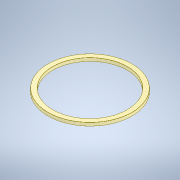
# Autodesk Inventor part: 201555-1-1-test
Saved by Autodesk Inventor 2021 (Build 250183000, 183)
## iProperties
Created: 2020-06-29
Part Number: 201555-1-1-test
Material: Nylon 6/6
Document SubType Name: Modeling
Density: 1.13 g/cm^3
Appearance: Nylon 6
Mass: 19.7025 g
Surface Area: 104.615 cm^2
Volume: 17.4358 cm^3
Author: MK
Subject: 100/120*5
Autodesk Inventor part; units mm, degrees
ref_plane "YZ Plane" through (0, 0, 0) normal (1, 0, 0) x (0, 1, 0)
ref_plane "XZ Plane" through (0, 0, 0) normal (0, 1, 0) x (-1, 0, 0)
ref_plane "XY Plane" through (0, 0, 0) normal (0, 0, 1) x (1, 0, 0)
sketch "Sketch1" plane through (0, 0, 0) normal (0, 0, 1) x (1, 0, 0)
  line L0 (115.2, 5.1) -> (129.8, 5.1)
  line L1 (129.8, 5.1) -> (129.8, -5.1)
  line L2 (129.8, -5.1) -> (115.2, -5.1)
  line L3 (115.2, -5.1) -> (115.2, 5.1)
  line L4 (0, 4.5532) -> (0, -4.5532)
  point P0 (0, 0)
  point P1 (0, 0)
  point P2 (115.2, 0)
  dimension "fascia_parameter" = 14.6
  dimension "height_parameter" = 10.2
  dimension "externalDiameter_parameter" = 259.6
  dimension "d5" = 230.4
  constraints: 10 end point, 2 coincident, 2 midpoint, 2 parallel, 1 horizontal, 1 horizontal alignment, 1 perpendicular, 1 vertical
  measures "fascia_parameter" distance of L0.start L0.end
  measures "height_parameter" distance of L0.end L1.end
  measures "externalDiameter_parameter" diameter of L1 L4
  measures "d5" diameter of L3 L4
revolve "Revolution1" add sketch "Sketch1" angle 360 about axis through (0, 4.5532, 0) along (0, -1, 0)
fillet "Fillet1" radius 0.3 4 edges at (-115.2, 5.1, 0) (-115.2, -5.1, 0) (-129.8, 5.1, 0) (-129.8, -5.1, 0)
body "Solid1"
